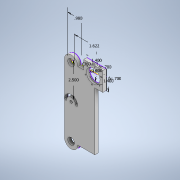
# Autodesk Inventor part: new conveyor bar
Saved by Autodesk Inventor 2021 (Build 250183000, 183)
## iProperties
Created: 2021-01-23
Part Number: new conveyor bar
Material: Generic
Document SubType Name: Modeling
Designer: User
Density: 1 g/cm^3
Appearance: Default
Author: User
Autodesk Inventor part; units mm, degrees
ref_plane "YZ Plane" through (0, 0, 0) normal (1, 0, 0) x (0, 1, 0)
ref_plane "XZ Plane" through (0, 0, 0) normal (0, 1, 0) x (-1, 0, 0)
ref_plane "XY Plane" through (0, 0, 0) normal (0, 0, 1) x (1, 0, 0)
sketch "Sketch1" plane through (0, 0, 0) normal (0, 0, 1) x (1, 0, 0)
  line L0 (0, -103.3729) -> (0, 23.6271) construction
  line L1 (-12.446, -103.3729) -> (-12.446, 23.6271)
  line L2 (12.446, 23.6271) -> (12.446, -103.3729)
  arc A0 (-12.446, -103.3729) -> (12.446, -103.3729) centre (0, -103.3729) ccw
  arc A1 (12.446, 23.6271) -> (-12.446, 23.6271) centre (0, 23.6271) ccw
  point P0 (0, 0)
  point P1 (0, -39.8729)
  dimension "d0" = 63.5
  dimension "d1" = 24.892
  constraints: 8 end point, 4 point on circle, 4 tangent, 2 centre point, 1 midpoint, 1 parallel, 1 vertical
  measures "d0" distance of point (0, -39.873) L0.end
  measures "d1" distance between parallel lines of L2 L1
extrude "Extrusion1" add sketch "Sketch1" along normal blind 6.096
sketch "Sketch2" plane through (0, 0, 6.096) normal (0, 0, 1) x (1, 0, 0)
  line L0 (-12.446, 23.6271) -> (-12.446, -103.3729) projected
  arc A0 (-12.446, -103.3729) -> (12.446, -103.3729) centre (0, -103.3729) ccw projected
  line L1 (12.446, -103.3729) -> (12.446, 23.6271) projected
  arc A1 (12.446, 23.6271) -> (-12.446, 23.6271) centre (0, 23.6271) ccw projected
  point P0 (0, 0)
  point P1 (0, -39.8729)
hole "Hole1" at (0, 23.6271, 6.096) at (0, -103.3729, 6.096) direction (0, 0, -1) diameter 12.446 depth 5.7785 tip angle 118
hole "Hole2" at (0, -39.8729, 0) direction (0, 0, 1) diameter 5.08 depth 5.7785 tip angle 118
sketch "Sketch3" plane through (0, 0, 0) normal (0, 0, -1) x (-1, 0, 0)
  circle A0 centre (0, -39.8729) radius 2.0116 projected
  arc A1 (10, -39.8729) -> (-10, -39.8729) centre (0, -39.8729) ccw construction
  arc A2 (12.032, -39.8729) -> (-12.032, -39.8729) centre (0, -39.8729) ccw
  arc A3 (7.968, -39.8729) -> (-7.968, -39.8729) centre (0, -39.8729) ccw
  arc A4 (7.968, -39.8729) -> (12.032, -39.8729) centre (10, -39.8729) ccw
  arc A5 (-12.032, -39.8729) -> (-7.968, -39.8729) centre (-10, -39.8729) ccw
  point P0 (0, 0)
  dimension "d18" = 2.032
  dimension "d19" = 10
  constraints: 10 point on circle, 5 centre point, 4 tangent, 1 coincident
  measures "d18" radius of A5
  measures "d19" distance of A1.centre A1.end
extrude "Extrusion2" cut sketch "Sketch3" against normal through all contours A4 A3 A5 A2
sketch "Sketch4" plane through (12.446, -103.3729, 0) normal (1, 0, 0) x (0, 0, -1)
  line L0 (0, 0) -> (0, 127) projected
  line L1 (0, 127) -> (-6.096, 127) projected
  line L2 (-6.096, 0) -> (-6.096, 127) projected
  line L3 (0, 0) -> (-6.096, 0) projected
  point P0 (0, 103.3729)
extrude "Extrusion3" add sketch "Sketch4" along normal blind 31.75
sketch "Sketch5" plane through (0, 0, 0) normal (0, 0, -1) x (-1, 0, 0)
  line L0 (-23.4086, 4.8323) -> (-58.9686, 4.8323)
  line L1 (-58.9686, 4.8323) -> (-58.9686, 40.3923)
  line L2 (-58.9686, 40.3923) -> (-23.4086, 40.3923)
  line L3 (-23.4086, 40.3923) -> (-23.4086, 4.8323)
  circle A0 centre (-41.1886, 22.6123) radius 12.7
  line L4 (8.5245, 22.6123) -> (-42.691, 22.6123)
  line L5 (-12.446, 23.6271) -> (-44.196, 23.6271) projected
  circle A1 centre (0, 23.6271) radius 5.6946 projected
  point P0 (0, 0)
  point P1 (-29.3576, 32.6261)
  point P2 (-43.9453, 37.8652)
  point P3 (-55.7764, 27.8514)
  point P4 (-53.0197, 12.5985)
  point P5 (-38.432, 7.3594)
  point P6 (-26.6009, 17.3732)
  point P7 (-47.5832, 13.0873)
  point P8 (-42.5032, 13.0873)
  point P9 (-28.4886, 22.6123)
  point P10 (-23.4086, 22.6123)
  dimension "d24" = 35.56
  dimension "d25" = 35.56
  dimension "d26" = 25.4
  dimension "d27" = 17.78
  dimension "d28" = 17.78
  dimension "d29" = 15.5
  dimension "d32" = 360
  dimension "d45" = 41.1886
  constraints: 8 end point, 2 parallel, 1 centre point, 1 horizontal, 1 perpendicular, 1 point on line, 1 vertical, 10 other
  measures "d24" distance of L1.end L2.end
  measures "d25" distance of L0.end L1.end
  measures "d26" diameter of A0
  measures "d27" distance from line of L2 A0.centre
  measures "d28" distance from line of L1 A0.centre
  measures "d29" distance of A0.centre point (-29.358, 32.626)
  measures "d45" horizontal distance of A0.centre A1.centre
extrude "Extrusion4" add sketch "Sketch5" against normal up to surface (6.096 mm away) contours L0 L1 L2 L3 L5 A0 L4 | L4 A0 L5 L3 | A0
extrude "Extrusion5" cut sketch "Sketch5" against normal through all contours A0
hole "Hole3" at (26.6009, 17.3732, 0) at (38.432, 7.3594, 0) at (53.0197, 12.5985, 0) at (55.7764, 27.8514, 0) at (43.9453, 37.8652, 0) at (29.3576, 32.6261, 0) direction (0, 0, 1) diameter 2.3368 depth 5.7785 tip angle 118
equation "\"d27\" = 0.5 * d25"
equation "\"d28\" = 0.5 * d24"
body "Solid1"
